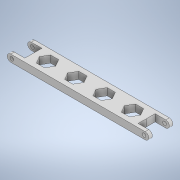
# Autodesk Inventor part: supportPiece
Saved by Autodesk Inventor 2021.2 (Build 252289000, 289)
## iProperties
Created: 2020-05-27
Part Number: supportPiece
Material: Generic
Document SubType Name: Modeling
Designer: robst
Density: 1 g/cm^3
Appearance: Default
Author: robst
Autodesk Inventor part; units mm, degrees
ref_plane "YZ Plane" through (0, 0, 0) normal (1, 0, 0) x (0, 1, 0)
ref_plane "XZ Plane" through (0, 0, 0) normal (0, 1, 0) x (-1, 0, 0)
ref_plane "XY Plane" through (0, 0, 0) normal (0, 0, 1) x (1, 0, 0)
sketch "Sketch1" plane through (0, 0, 0) normal (0, 1, 0) x (-1, 0, 0)
  line L0 (63.5003, 10.795) -> (-63.5003, 10.795)
  line L1 (-63.5, -10.795) -> (63.5, -10.795)
  line L2 (63.5003, 10.795) -> (-63.5, -10.795) construction
  line L3 (-63.5003, 10.795) -> (63.5, -10.795) construction
  line L4 (-63.5, -7.62) -> (-50.8, -7.62)
  line L5 (-50.8, -7.62) -> (-50.8, 0)
  line L6 (0, 0) -> (-63.5, -0.0014) construction
  line L7 (0, 0) -> (0, -10.795) construction
  line L8 (-63.5003, 7.6171) -> (-50.8003, 7.6177)
  line L9 (-50.8003, 7.6177) -> (-50.8, 0)
  line L10 (63.5, -7.62) -> (50.8, -7.62)
  line L11 (50.8, -7.62) -> (50.8, 0)
  line L12 (63.5003, 7.6171) -> (50.8003, 7.6177)
  line L13 (50.8003, 7.6177) -> (50.8, 0)
  line L14 (63.5, -10.795) -> (63.5, -7.62)
  line L15 (63.5003, 7.6171) -> (63.5003, 10.795)
  line L16 (-63.5003, 10.795) -> (-63.5003, 7.6171)
  line L17 (-63.5, -7.62) -> (-63.5, -10.795)
  dimension "length" = 127
  dimension "oneHalfCutoffWidth" = 7.62
  dimension "cutoutWidth" = 12.7
  dimension "width" = 21.59
  constraints: 36 end point, 7 symmetric about line, 6 parallel, 2 perpendicular, 2 point on line, 1 horizontal, 1 midpoint, 1 vertical
  measures "length" distance of L1.start L1.end
  measures "oneHalfCutoffWidth" distance from line of L4 L6.start
  measures "cutoutWidth" distance of L4.start L4.end
  measures "width" distance from line of L0 L7.end
extrude "Extrusion1" add sketch "Sketch1" along normal mid plane 6.35
sketch "Sketch2" plane through (-63.5003, 3.175, 10.795) normal (0, 0, 1) x (1, 0, 0)
  line L0 (63.5003, -3.175) -> (63.5003, 0) construction
  line L1 (0, 0) -> (127.0007, 0) construction
  point P0 (122.8347, -3.175)
  point P1 (4.1659, -3.175)
  dimension "d8" = 59.3344
  constraints: 2 end point, 1 midpoint, 1 symmetric about line
  measures "d8" distance of point (122.835, -3.175) L0.start
hole "Hole1" at (59.3344, 0, 10.795) at (-59.3344, 0, 10.795) direction (0, 0, -1) diameter 3.2766 end through all clearance for "Flat Head Machine Screw (82)" size "#4" standard "Ansi Unified Screw Threads"
fillet "Fillet2" radius 3.175 8 edges at (63.5, 3.175, -9.2075) (63.5, -3.175, -9.2075) (63.5003, 3.175, 9.2061) (63.5003, -3.175, 9.2061) (-63.5003, 3.175, 9.2061) (-63.5003, -3.175, 9.2061) (-63.5, 3.175, -9.2075) (-63.5, -3.175, -9.2075)
sketch "Sketch5" plane through (0, 3.175, 0) normal (0, 1, 0) x (1, 0, 0)
  line L0 (-50.8, 0) -> (50.8, 0) construction
  line L1 (-34.4338, 6.35) -> (-30.7677, 0)
  line L2 (-30.7677, 0) -> (-34.4338, -6.35)
  line L3 (-34.4338, -6.35) -> (-41.7662, -6.35)
  line L4 (-41.7662, -6.35) -> (-45.4323, 0)
  line L5 (-45.4323, 0) -> (-41.7662, 6.35)
  line L6 (-41.7662, 6.35) -> (-34.4338, 6.35)
  line L7 (-50.8, 0) -> (-50.8003, -7.6177) projected
  line L8 (-16.3662, 6.35) -> (-9.0338, 6.35)
  line L9 (-9.0338, 6.35) -> (-5.3677, 0)
  line L10 (-5.3677, 0) -> (-9.0338, -6.35)
  line L11 (-9.0338, -6.35) -> (-16.3662, -6.35)
  line L12 (-16.3662, -6.35) -> (-20.0323, 0)
  line L13 (-20.0323, 0) -> (-16.3662, 6.35)
  line L14 (9.0338, 6.35) -> (16.3662, 6.35)
  line L15 (16.3662, 6.35) -> (20.0323, 0)
  line L16 (20.0323, 0) -> (16.3662, -6.35)
  line L17 (16.3662, -6.35) -> (9.0338, -6.35)
  line L18 (9.0338, -6.35) -> (5.3677, 0)
  line L19 (5.3677, 0) -> (9.0338, 6.35)
  line L20 (34.4338, 6.35) -> (41.7662, 6.35)
  line L21 (41.7662, 6.35) -> (45.4323, 0)
  line L22 (45.4323, 0) -> (41.7662, -6.35)
  line L23 (41.7662, -6.35) -> (34.4338, -6.35)
  line L24 (34.4338, -6.35) -> (30.7677, 0)
  line L25 (30.7677, 0) -> (34.4338, 6.35)
  point P0 (0, 0)
  point P1 (-38.1, 0)
  dimension "d18" = 12.7
  dimension "d19" = 12.7
  dimension "d22" = 25.4
  constraints: 50 end point, 3 horizontal, 1 point on line, 49 other
  measures "d18" distance between parallel lines of L3 L6
  measures "d19" distance from line of point (-38.1, 0) L7
  measures "d22" distance of L5.end L8.start
extrude "Extrusion2" cut sketch "Sketch5" against normal through all
equation "\"endFilet\" = 0.5 * depth"
equation "\"depth\" = 6.35"
body "Solid1"
